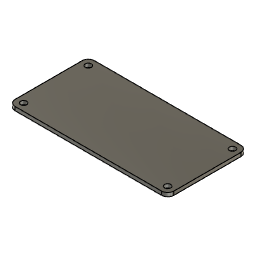
Platform_ general (Autodesk Fusion 360 design; units mm, degrees)
Autodesk Fusion 360 part; units mm, degrees
note: some values were not read from the file. Set by a fixed rule: which sketch regions a step uses.
sketch "Sketch1" plane through (0, 0, 0) normal (0, 0, 1) x (1, 0, 0)
  line L0 (-60, 32.5) -> (0, 32.5)
  line L1 (0, -32.5) -> (-60, -32.5)
  line L2 (-65, -27.5) -> (-65, 27.5)
  arc A0 (-60, 32.5) -> (-65, 27.5) centre (-60, 27.5) ccw
  arc A1 (-65, -27.5) -> (-60, -32.5) centre (-60, -27.5) ccw
  circle A2 centre (-59, 26.5) radius 2.5
  circle A3 centre (-59, -26.5) radius 2.5
  line L3 (0, 32.5) -> (0, -32.5) construction
  line L4 (65, -27.5) -> (65, 27.5)
  circle A4 centre (59, 26.5) radius 2.5
  arc A5 (60, -32.5) -> (65, -27.5) centre (60, -27.5) ccw
  circle A6 centre (59, -26.5) radius 2.5
  arc A7 (65, 27.5) -> (60, 32.5) centre (60, 27.5) ccw
  line L5 (0, -32.5) -> (60, -32.5)
  line L6 (60, 32.5) -> (0, 32.5)
  dimension "d1" = 65
  dimension "d3" = 32.5
  dimension "d4" = 32.5
  dimension "d5" = 5
  dimension "d6" = 5
  dimension "d9" = 5
  dimension "d10" = 6
  dimension "d11" = 6
  dimension "d12" = 5
  dimension "d13" = 6
  dimension "d14" = 6
  dimension "d35" = 65
  dimension "d36" = 65
  constraint horizontal L0
  constraint horizontal L1
  constraint vertical L2
  constraint tangent L0 A0
  constraint tangent L2 A0
  constraint tangent L1 A1
  constraint tangent L2 A1
  constraint symmetric L0.start L3 A7.end
  constraint symmetric L2.end L3 L4.end
  constraint symmetric A0 L3 A7
  constraint symmetric L1.end L3 A5.start
  measures "d1" distance of origin L2
  measures "d3" distance of origin L0
  measures "d4" distance of origin L1
  measures "d5" radius of A0
  measures "d6" radius of A1
  measures "d9" diameter of A2
  measures "d10" distance of L0 A2.centre
  measures "d11" distance of L2 A2.centre
  measures "d12" diameter of A3
  measures "d13" distance of L1 A3.centre
  measures "d14" distance of L2 A3.centre
  measures "d35" distance of L2 L0.end
  measures "d36" distance of L2 L1.start
extrude "Extrude4" add sketch "Sketch1" along normal blind 3
equation "d3 = ( 65 / 2 ) * 1 mm"
equation "d4 = d3"
equation "d6 = d5"
equation "d11 = d10"
equation "d12 = d9"
equation "d13 = d10"
equation "d14 = d10"
equation "d35 = d1"
equation "d36 = d1"
